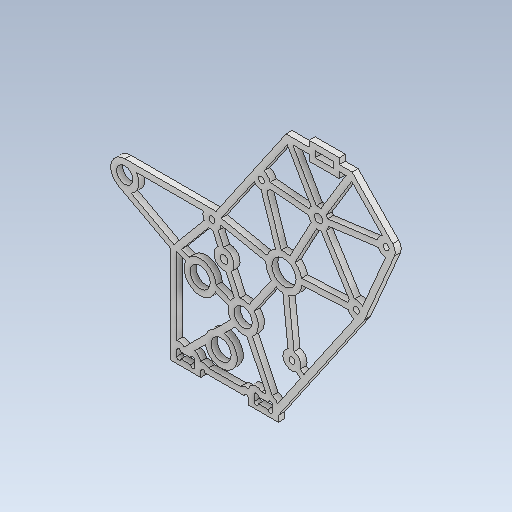
# Autodesk Inventor part: 横回転首振りフレーム２
Saved by Autodesk Inventor 2020 (Build 240168000, 168)
## iProperties
Created: 2020-02-26
Part Number: 横回転首振りフレーム２
Material: アルミニウム 2014-T4
Document SubType Name: Modeling
Designer: tanjihayato
Density: 2.8 g/cm^3
Appearance: サテン
Mass: 28.1218 g
Surface Area: 128.912 cm^2
Volume: 10.0435 cm^3
Author: tanjihayato
Autodesk Inventor part; units mm, degrees
ref_plane "YZ Plane" through (0, 0, 0) normal (1, 0, 0) x (0, 1, 0)
ref_plane "XZ Plane" through (0, 0, 0) normal (0, 1, 0) x (-1, 0, 0)
ref_plane "XY Plane" through (0, 0, 0) normal (0, 0, 1) x (1, 0, 0)
sketch "スケッチ1" plane through (0, 0, 0) normal (0, 0, 1) x (1, 0, 0)
  circle A0 centre (-11.4931, -19.1593) radius 14 construction
  circle A1 centre (16.245, -15.3385) radius 14 construction
  line L0 (-170.915, -81.4118) -> (490.0044, -81.4118)
  line L1 (-197.2268, -33.1593) -> (179.6604, -33.1593) construction
  line L2 (-178.6504, 68.5882) -> (447.0756, 68.5882) construction
  circle A2 centre (-11.4931, -19.1593) radius 14 construction
  circle A3 centre (-21.8854, 6.8407) radius 14 construction
  circle A4 centre (-0.5211, 0.3031) radius 20.05 construction
  circle A5 centre (-0.5211, 0.3031) radius 22.3421 construction
  circle A6 centre (0, 0) radius 22.3421 construction
  circle A7 centre (-0.5211, 0.3031) radius 5.05 construction
  circle A8 centre (19.689, 29.6103) radius 30.55 construction
  circle A9 centre (19.689, 29.6103) radius 10.1 construction
  circle A10 centre (39.672, 58.5882) radius 25.1 construction
  line L3 (-0.5211, 0.3031) -> (39.672, 58.5882) construction
  circle A11 centre (39.672, 58.5882) radius 27.1 construction
  circle A12 centre (19.689, 29.6103) radius 31.55 construction
  circle A13 centre (19.689, 29.6103) radius 12.1 construction
  circle A14 centre (-0.5211, 0.3031) radius 20.55 construction
  circle A15 centre (-0.5211, 0.3031) radius 6.05 construction
  circle A16 centre (36.8436, 61.4166) radius 4 construction
  circle A17 centre (36.8436, 61.4166) radius 2
  line L4 (36.8436, 61.4166) -> (39.672, 58.5882)
  line L5 (39.672, 58.5882) -> (22.909, 61.4166) construction
  circle A18 centre (22.909, 61.4166) radius 2
  circle A19 centre (22.909, 61.4166) radius 5
  line L6 (28.2635, 50.4737) -> (31.5576, 69.9968) construction
  line L7 (31.5576, 69.9968) -> (51.0806, 66.7027) construction
  line L8 (51.0806, 66.7027) -> (47.7865, 47.1796) construction
  line L9 (47.7865, 47.1796) -> (28.2635, 50.4737) construction
  circle A20 centre (39.672, 58.5882) radius 9
  circle A21 centre (28.2635, 50.4737) radius 2.5
  circle A22 centre (47.7865, 47.1796) radius 2.5
  circle A23 centre (51.0806, 66.7027) radius 2.5
  circle A24 centre (31.5576, 69.9968) radius 2.5
  circle A25 centre (28.2635, 50.4737) radius 5
  line L10 (22.909, 61.4166) -> (36.8436, 61.4166) construction
  line L11 (-26.0808, 51.4166) -> (-426.0808, 51.4166)
  line L12 (-26.0808, 24.4166) -> (23.9192, 24.4166)
  circle A26 centre (39.672, 58.5882) radius 17.5
  circle A27 centre (47.7865, 47.1796) radius 2.1
  circle A28 centre (28.2635, 50.4737) radius 2.1
  circle A29 centre (31.5576, 69.9968) radius 2.1
  circle A30 centre (51.0806, 66.7027) radius 2.1
  circle A31 centre (47.7865, 47.1796) radius 5
  circle A32 centre (31.5576, 69.9968) radius 5
  circle A33 centre (51.0806, 66.7027) radius 5
  circle A34 centre (39.672, 58.5882) radius 19.5
  circle A35 centre (39.672, 58.5882) radius 20.5
  line L13 (20.7504, 89.6882) -> (53.4998, 89.6882)
  line L14 (53.4998, 89.6882) -> (73.6516, 68.9857)
  line L15 (20.7504, 89.6882) -> (-13.977, 39.0272)
  circle A36 centre (-59.2702, 32.0272) radius 5.025 construction
  circle A37 centre (-59.2702, 32.0272) radius 4
  arc A38 (-59.2702, 39.0272) -> (-62.5897, 25.8643) centre (-59.2702, 32.0272) ccw
  line L16 (-59.2702, 39.0272) -> (-13.977, 39.0272)
  line L17 (-62.5897, 25.8643) -> (-36.5547, 11.8407)
  line L18 (-36.5547, 11.8407) -> (-36.5547, -33.1593)
  arc A39 (74.5655, 64.0796) -> (73.6516, 68.9857) centre (70.4271, 65.8469) ccw
  circle A40 centre (8.5193, 63.8863) radius 4.5 construction
  arc A41 (59.4085, 28.8085) -> (59.8353, 29.5856) centre (55.6969, 31.3528) ccw
  circle A42 centre (23.6647, -6.2198) radius 4.5
  circle A43 centre (-16.0241, 34.5272) radius 4.5 construction
  line L19 (59.8353, 29.5856) -> (74.5655, 64.0796)
  line L20 (32.172, 89.6882) -> (32.172, 92.6882)
  line L21 (32.172, 92.6882) -> (47.172, 92.6882)
  line L22 (47.172, 92.6882) -> (47.172, 89.6882)
  line L23 (35.172, 89.6882) -> (35.172, 86.6882)
  line L24 (35.172, 86.6882) -> (44.172, 86.6882)
  line L25 (44.172, 86.6882) -> (44.172, 89.6882)
  circle A44 centre (70.4271, 65.8469) radius 1.5
  circle A45 centre (55.6969, 31.3528) radius 1.5
  circle A46 centre (23.6647, -6.2198) radius 1.5
  circle A47 centre (-16.0241, 34.5272) radius 1.5
  circle A48 centre (8.5193, 63.8863) radius 1.5
  circle A49 centre (-10.0662, 20.4166) radius 4 construction
  circle A50 centre (-10.0662, 20.4166) radius 2
  line L26 (1.9305, -36.1593) -> (16.9305, -36.1593)
  line L27 (16.9305, -36.1593) -> (16.9305, -33.1593)
  line L28 (1.9305, -33.1593) -> (1.9305, -36.1593)
  arc A51 (1.9305, -33.1593) -> (-0.1695, -33.1593) centre (0.8805, -33.1593) ccw
  line L29 (13.9305, -30.1593) -> (13.9305, -33.1593)
  arc A52 (13.9305, -30.1593) -> (11.8305, -30.1593) centre (12.8805, -30.1593) ccw
  line L30 (7.0305, -30.1593) -> (11.8305, -30.1593)
  arc A53 (7.0305, -30.1593) -> (4.9305, -30.1593) centre (5.9805, -30.1593) ccw
  line L31 (4.9305, -33.1593) -> (4.9305, -30.1593)
  arc A54 (4.9305, -33.1593) -> (7.0305, -33.1593) centre (5.9805, -33.1593) ccw
  arc A55 (11.8305, -33.1593) -> (13.9305, -33.1593) centre (12.8805, -33.1593) ccw
  line L32 (-36.5547, -36.1593) -> (-21.5547, -36.1593)
  line L33 (-21.5547, -36.1593) -> (-21.5547, -33.1593)
  arc A56 (-19.4547, -33.1593) -> (-21.5547, -33.1593) centre (-20.5047, -33.1593) ccw
  line L34 (-36.5547, -33.1593) -> (-36.5547, -36.1593)
  arc A57 (-33.5547, -33.1593) -> (-31.4547, -33.1593) centre (-32.5047, -33.1593) ccw
  line L35 (-33.5547, -33.1593) -> (-33.5547, -30.1593)
  arc A58 (-31.4547, -30.1593) -> (-33.5547, -30.1593) centre (-32.5047, -30.1593) ccw
  line L36 (-31.4547, -30.1593) -> (-26.6547, -30.1593)
  arc A59 (-24.5547, -30.1593) -> (-26.6547, -30.1593) centre (-25.6047, -30.1593) ccw
  line L37 (-24.5547, -30.1593) -> (-24.5547, -33.1593)
  arc A60 (-26.6547, -33.1593) -> (-24.5547, -33.1593) centre (-25.6047, -33.1593) ccw
  line L38 (59.4085, 28.8085) -> (16.9305, -33.1593)
  circle A61 centre (-21.8854, 6.8407) radius 5
  circle A62 centre (-11.4931, -19.1593) radius 5
  line L39 (-31.4547, -33.1593) -> (-26.6547, -33.1593)
  line L40 (-19.4547, -33.1593) -> (-0.1695, -33.1593)
  line L41 (7.0305, -33.1593) -> (11.8305, -33.1593)
  line L42 (0.4485, -25.8914) -> (-27.1419, -10.3373) construction
  line L43 (-27.1419, -10.3373) -> (-17.3768, 21.5744) construction
  circle A63 centre (-21.8854, 6.8407) radius 8
  circle A64 centre (-11.4931, -19.1593) radius 8
  circle A65 centre (-19.5445, 14.4905) radius 1.3
  circle A66 centre (-24.2262, -0.8092) radius 1.3
  circle A67 centre (-18.4619, -15.2306) radius 1.3
  circle A68 centre (-4.5242, -23.088) radius 1.3
  circle A69 centre (-0.5211, 0.3031) radius 4.5
  circle A70 centre (19.689, 29.6103) radius 6
  arc A71 (87.3323, 12.0445) -> (87.1264, 18.8999) centre (85.1711, 15.4104) ccw
  line L44 (16.9305, -33.1593) -> (87.3323, 12.0445)
  line L45 (87.1264, 18.8999) -> (61.4227, 33.3027)
  circle A72 centre (85.1711, 15.4104) radius 2
  dimension "d0" = 150
  dimension "d1" = 28
  dimension "d2" = 28
  dimension "d3" = 40.1
  dimension "d4" = 10.1
  dimension "d5" = 61.1
  dimension "d6" = 20.2
  dimension "d7" = 50.2
  dimension "d8" = 10
  dimension "d9" = 2
  dimension "d10" = 1
  dimension "d11" = 2
  dimension "d12" = 0.5
  dimension "d13" = 1
  dimension "d14" = 40
  dimension "d15" = 8
  dimension "d16" = 4
  dimension "d17" = 4
  dimension "d18" = 45
  dimension "d19" = 17
  dimension "d20" = 4
  dimension "d21" = 3
  dimension "d22" = 1
  dimension "d23" = 5
  dimension "d24" = 5
  dimension "d25" = 5
  dimension "d26" = 5
  dimension "d27" = 10
  dimension "d28" = 400
  dimension "d29" = 10
  dimension "d30" = 50
  dimension "d31" = 50
  dimension "d32" = 27
  dimension "d33" = 27
  dimension "d34" = 35
  dimension "d35" = 4.2
  dimension "d36" = 4.2
  dimension "d37" = 4.2
  dimension "d38" = 4.2
  dimension "d39" = 10
  dimension "d40" = 10
  dimension "d41" = 10
  dimension "d42" = 2
  dimension "d43" = 1
  dimension "d44" = 8
  dimension "d45" = 3
  dimension "d46" = 4
  dimension "d47" = 9
  dimension "d48" = 9
  dimension "d49" = 9
  dimension "d50" = 9
  dimension "d51" = 9
  dimension "d52" = 3
  dimension "d53" = 15
  dimension "d54" = 3
  dimension "d55" = 9
  dimension "d56" = 3
  dimension "d57" = 7.5
  dimension "d58" = 3
  dimension "d59" = 3
  dimension "d60" = 3
  dimension "d61" = 3
  dimension "d62" = 3
  dimension "d63" = 8
  constraints: 90 end point, 71 centre point, 34 point on circle, 32 coincident, 23 tangent, 12 point on line, 7 perpendicular, 6 horizontal, 3 parallel, 1 collinear, 1 equal radius, 1 vertical, 22 other
  measures "d0" distance between parallel lines of L0 L2
  measures "d1" diameter of A2
  measures "d2" diameter of A3
  measures "d3" diameter of A4
  measures "d4" diameter of A7
  measures "d5" diameter of A8
  measures "d6" diameter of A9
  measures "d7" diameter of A10
  measures "d8" distance from line of L2 L3.end
  measures "d10" radial gap between concentric circles of A8 A12
  measures "d11" radial gap between concentric circles of A9 A13
  measures "d12" radial gap between concentric circles of A4 A14
  measures "d13" radial gap between concentric circles of A7 A15
  measures "d15" diameter of A16
  measures "d16" diameter of A17
  measures "d17" distance of A16.centre L3.end
  measures "d18" angle of L0 L4
  measures "d19" distance of L3.end L5.end
  measures "d20" diameter of A18
  measures "d21" radial gap between concentric circles of A18 A19
  measures "d23" diameter of A21
  measures "d24" diameter of A22
  measures "d25" diameter of A23
  measures "d26" diameter of A24
  measures "d27" diameter of A25
  measures "d28" distance of L11.start L11.end
  measures "d29" distance between parallel lines of L10 L11
  measures "d30" distance of L5.end L11.start
  measures "d31" distance of L12.start L12.end
  measures "d32" distance between parallel lines of L12 L11
  measures "d33" distance of L11.start L12.start
  measures "d34" diameter of A26
  measures "d35" diameter of A27
  measures "d36" diameter of A28
  measures "d37" diameter of A29
  measures "d38" diameter of A30
  measures "d39" diameter of A31
  measures "d40" diameter of A32
  measures "d41" diameter of A33
  measures "d42" radial gap between concentric circles of A26 A34
  measures "d43" radial gap between concentric circles of A34 A35
  measures "d44" diameter of A37
  measures "d45" radial gap between concentric circles of A37 A38
  measures "d47" diameter of A39
  measures "d48" diameter of A40
  measures "d49" diameter of A41
  measures "d50" diameter of A42
  measures "d51" diameter of A43
  measures "d52" distance of L20.start L20.end
  measures "d53" distance of L20.end L21.end
  measures "d54" distance of L23.start L23.end
  measures "d55" distance of L23.end L24.end
  measures "d56" distance between parallel lines of L22 L25
  measures "d57" distance from line of L3.end L20
  measures "d58" diameter of A44
  measures "d59" diameter of A45
  measures "d60" diameter of A46
  measures "d61" diameter of A47
  measures "d62" diameter of A48
  measures "d63" diameter of A49
extrude "押し出し1" add sketch "スケッチ1" along normal blind 3 contours A18 A26 | A18 A26 A19 | A26 A18 | A18 A26 A19 A34 | A26 A32 A20 A25 A19 | A19 A34 A26 A25 A31 A33 A32 | A34 A19 A35 | A19 A35 A34 | A32 A26 | A26 A32 | A26 A25 | A25 A26 | A35 A19 | A26 A33 A20 A32 | A20 | A20 A31 A26 A25 | A33 A26 | A26 A33 | A33 A26 A31 A20 | A31 A26 | A26 A31 | A21 | A22 | A23 | A24 | A27 | A28 | A29 | A30 | L13 L23 L24 L25 L14 A39 L19 A41 L38 L27 L26 L28 A51 L40 A56 L33 L32 L34 L18 L17 A38 L16 L15 | L20 L21 L22 L13 | A42 | A63 A66 A65 | A65 A63 | A63 A65 | A66 A63 | A63 A66 | A64 A68 A67 | A67 A64 | A64 A67 | A68 A64 | A64 A68
sketch "スケッチ2" plane through (0, 0, 3) normal (0, 0, 1) x (1, 0, 0)
  line L0 (-13.977, 39.0272) -> (-59.2702, 39.0272) projected
  arc A0 (-59.2702, 39.0272) -> (-62.5897, 25.8643) centre (-59.2702, 32.0272) ccw projected
  line L1 (-62.5897, 25.8643) -> (-36.5547, 11.8407) projected
  line L2 (-36.5547, 11.8407) -> (-36.5547, -36.1593) projected
  line L3 (-36.5547, -36.1593) -> (-21.5547, -36.1593) projected
  line L4 (-21.5547, -36.1593) -> (-21.5547, -33.1593) projected
  arc A1 (-19.4547, -33.1593) -> (-21.5547, -33.1593) centre (-20.5047, -33.1593) ccw projected
  line L5 (-19.4547, -33.1593) -> (-0.1695, -33.1593) projected
  arc A2 (1.9305, -33.1593) -> (-0.1695, -33.1593) centre (0.8805, -33.1593) ccw projected
  line L6 (1.9305, -33.1593) -> (1.9305, -36.1593) projected
  line L7 (1.9305, -36.1593) -> (16.9305, -36.1593) projected
  line L8 (16.9305, -36.1593) -> (16.9305, -33.1593) projected
  line L9 (16.9305, -33.1593) -> (59.4085, 28.8085) projected
  arc A3 (59.4085, 28.8085) -> (59.8353, 29.5856) centre (55.6969, 31.3528) ccw projected
  line L10 (59.8353, 29.5856) -> (74.5655, 64.0796) projected
  arc A4 (74.5655, 64.0796) -> (73.6516, 68.9857) centre (70.4271, 65.8469) ccw projected
  line L11 (73.6516, 68.9857) -> (53.4998, 89.6882) projected
  line L12 (53.4998, 89.6882) -> (47.172, 89.6882) projected
  line L13 (47.172, 89.6882) -> (47.172, 92.6882) projected
  line L14 (47.172, 92.6882) -> (32.172, 92.6882) projected
  line L15 (32.172, 92.6882) -> (32.172, 89.6882) projected
  line L16 (32.172, 89.6882) -> (20.7504, 89.6882) projected
  line L17 (20.7504, 89.6882) -> (-13.977, 39.0272) projected
  circle A5 centre (36.8436, 61.4166) radius 2 projected
  arc A6 (-26.6547, -33.1593) -> (-24.5547, -33.1593) centre (-25.6047, -33.1593) ccw projected
  line L18 (-26.6547, -33.1593) -> (-31.4547, -33.1593) projected
  arc A7 (-33.5547, -33.1593) -> (-31.4547, -33.1593) centre (-32.5047, -33.1593) ccw projected
  line L19 (-33.5547, -33.1593) -> (-33.5547, -30.1593) projected
  arc A8 (-31.4547, -30.1593) -> (-33.5547, -30.1593) centre (-32.5047, -30.1593) ccw projected
  line L20 (-31.4547, -30.1593) -> (-26.6547, -30.1593) projected
  arc A9 (-24.5547, -30.1593) -> (-26.6547, -30.1593) centre (-25.6047, -30.1593) ccw projected
  line L21 (-24.5547, -30.1593) -> (-24.5547, -33.1593) projected
  line L22 (13.9305, -30.1593) -> (13.9305, -33.1593) projected
  arc A10 (11.8305, -33.1593) -> (13.9305, -33.1593) centre (12.8805, -33.1593) ccw projected
  line L23 (11.8305, -33.1593) -> (7.0305, -33.1593) projected
  arc A11 (4.9305, -33.1593) -> (7.0305, -33.1593) centre (5.9805, -33.1593) ccw projected
  line L24 (4.9305, -33.1593) -> (4.9305, -30.1593) projected
  arc A12 (7.0305, -30.1593) -> (4.9305, -30.1593) centre (5.9805, -30.1593) ccw projected
  line L25 (7.0305, -30.1593) -> (11.8305, -30.1593) projected
  arc A13 (13.9305, -30.1593) -> (11.8305, -30.1593) centre (12.8805, -30.1593) ccw projected
  circle A14 centre (8.5193, 63.8863) radius 1.5 projected
  circle A15 centre (-59.2702, 32.0272) radius 4 projected
  circle A16 centre (-0.5211, 0.3031) radius 4.5 projected
  circle A17 centre (-16.0241, 34.5272) radius 1.5 projected
  circle A18 centre (70.4271, 65.8469) radius 1.5 projected
  circle A19 centre (55.6969, 31.3528) radius 1.5 projected
  circle A20 centre (-10.0662, 20.4166) radius 2 projected
  circle A21 centre (19.689, 29.6103) radius 6 projected
  line L26 (35.172, 89.6882) -> (44.172, 89.6882) projected
  line L27 (44.172, 89.6882) -> (44.172, 86.6882) projected
  line L28 (44.172, 86.6882) -> (35.172, 86.6882) projected
  line L29 (35.172, 86.6882) -> (35.172, 89.6882) projected
  circle A22 centre (-11.4931, -19.1593) radius 5 projected
  circle A23 centre (-21.8854, 6.8407) radius 5 projected
  circle A24 centre (23.6647, -6.2198) radius 1.5 projected
  line L30 (22.3311, 86.6882) -> (35.172, 86.6882)
  line L31 (35.172, 86.6882) -> (35.172, 89.6882)
  line L32 (35.172, 89.6882) -> (44.172, 89.6882)
  line L33 (44.172, 89.6882) -> (44.172, 86.6882)
  line L34 (44.172, 86.6882) -> (52.2334, 86.6882)
  line L35 (52.2334, 86.6882) -> (71.5019, 66.8931)
  arc A25 (71.8065, 65.2578) -> (71.5019, 66.8931) centre (70.4271, 65.8469) ccw
  line L36 (71.8065, 65.2578) -> (57.0763, 30.7638)
  arc A26 (56.9341, 30.5047) -> (57.0763, 30.7638) centre (55.6969, 31.3528) ccw
  line L37 (56.9341, 30.5047) -> (13.9305, -32.2298)
  line L38 (13.9305, -32.2298) -> (13.9305, -33.1593)
  line L39 (13.9305, -33.1593) -> (4.9305, -33.1593)
  arc A27 (4.9305, -33.1593) -> (-1.8402, -30.1593) centre (0.8805, -33.1593) ccw
  line L40 (-1.8402, -30.1593) -> (-17.7839, -30.1593)
  arc A28 (-17.7839, -30.1593) -> (-24.5547, -33.1593) centre (-20.5047, -33.1593) ccw
  line L41 (-24.5547, -33.1593) -> (-33.5547, -33.1593)
  line L42 (-33.5547, -33.1593) -> (-33.5547, 13.6322)
  line L43 (-33.5547, 13.6322) -> (-61.1671, 28.5055)
  arc A29 (-59.2702, 36.0272) -> (-61.1671, 28.5055) centre (-59.2702, 32.0272) ccw
  line L44 (-59.2702, 36.0272) -> (-12.3962, 36.0272)
  line L45 (-12.3962, 36.0272) -> (22.3311, 86.6882)
  line L46 (32.172, 83.6882) -> (47.172, 83.6882)
  line L47 (47.172, 83.6882) -> (47.172, 92.6882)
  line L48 (47.172, 92.6882) -> (32.172, 92.6882)
  line L49 (32.172, 92.6882) -> (32.172, 83.6882)
  circle A30 centre (8.5193, 63.8863) radius 4.5
  circle A31 centre (36.8436, 61.4166) radius 5
  circle A32 centre (70.4271, 65.8469) radius 4.5
  circle A33 centre (55.6969, 31.3528) radius 4.5
  circle A34 centre (19.689, 29.6103) radius 9
  circle A35 centre (23.6647, -6.2198) radius 4.5
  circle A36 centre (-0.5211, 0.3031) radius 7.5
  circle A37 centre (-11.4931, -19.1593) radius 8
  circle A38 centre (-21.8854, 6.8407) radius 8
  circle A39 centre (-10.0662, 20.4166) radius 5
  circle A40 centre (-16.0241, 34.5272) radius 4.5
  circle A41 centre (-59.2702, 32.0272) radius 7
  line L50 (10.1598, -27.1593) -> (8.7013, -27.1593)
  arc A42 (8.7013, -27.1593) -> (1.9305, -30.1593) centre (5.9805, -30.1593) ccw
  line L51 (1.9305, -30.1593) -> (1.9305, -33.1593)
  arc A43 (1.9305, -33.1593) -> (8.7013, -36.1593) centre (5.9805, -33.1593) ccw
  line L52 (8.7013, -36.1593) -> (10.1598, -36.1593)
  arc A44 (10.1598, -36.1593) -> (16.9305, -33.1593) centre (12.8805, -33.1593) ccw
  line L53 (16.9305, -33.1593) -> (16.9305, -30.1593)
  arc A45 (16.9305, -30.1593) -> (10.1598, -27.1593) centre (12.8805, -30.1593) ccw
  line L54 (-28.3254, -27.1593) -> (-29.7839, -27.1593)
  arc A46 (-29.7839, -27.1593) -> (-36.5547, -30.1593) centre (-32.5047, -30.1593) ccw
  line L55 (-36.5547, -30.1593) -> (-36.5547, -33.1593)
  arc A47 (-36.5547, -33.1593) -> (-29.7839, -36.1593) centre (-32.5047, -33.1593) ccw
  line L56 (-29.7839, -36.1593) -> (-28.3254, -36.1593)
  arc A48 (-28.3254, -36.1593) -> (-21.5547, -33.1593) centre (-25.6047, -33.1593) ccw
  line L57 (-21.5547, -33.1593) -> (-21.5547, -30.1593)
  arc A49 (-21.5547, -30.1593) -> (-28.3254, -27.1593) centre (-25.6047, -30.1593) ccw
  circle A50 centre (70.4271, 65.8469) radius 1.5 projected
  line L58 (36.8436, 61.4166) -> (70.4271, 65.8469) construction
  line L59 (37.0398, 59.9295) -> (70.6232, 64.3597)
  line L60 (70.2309, 67.334) -> (36.6474, 62.9037)
  arc A51 (36.6474, 62.9037) -> (37.0398, 59.9295) centre (36.8436, 61.4166) ccw
  arc A52 (70.6232, 64.3597) -> (70.2309, 67.334) centre (70.4271, 65.8469) ccw
  circle A53 centre (55.6969, 31.3528) radius 1.5 projected
  line L61 (55.6969, 31.3528) -> (36.8436, 61.4166) construction
  line L62 (56.9677, 32.1498) -> (38.1144, 62.2136)
  line L63 (35.5728, 60.6197) -> (54.4261, 30.5559)
  arc A54 (54.4261, 30.5559) -> (56.9677, 32.1498) centre (55.6969, 31.3528) ccw
  arc A55 (38.1144, 62.2136) -> (35.5728, 60.6197) centre (36.8436, 61.4166) ccw
  line L64 (8.5193, 63.8863) -> (36.8436, 61.4166) construction
  line L65 (8.389, 62.3919) -> (36.7133, 59.9223)
  line L66 (36.9739, 62.911) -> (8.6496, 65.3806)
  arc A56 (8.6496, 65.3806) -> (8.389, 62.3919) centre (8.5193, 63.8863) ccw
  arc A57 (36.7133, 59.9223) -> (36.9739, 62.911) centre (36.8436, 61.4166) ccw
  line L67 (52.2334, 86.6882) -> (36.8436, 61.4166) construction
  line L68 (50.9522, 87.4684) -> (35.5625, 62.1968)
  line L69 (38.1247, 60.6364) -> (53.5145, 85.908)
  arc A58 (53.5145, 85.908) -> (50.9522, 87.4684) centre (52.2334, 86.6882) ccw
  arc A59 (35.5625, 62.1968) -> (38.1247, 60.6364) centre (36.8436, 61.4166) ccw
  line L70 (22.3311, 86.6882) -> (36.8436, 61.4166) construction
  line L71 (21.0304, 85.9412) -> (35.5428, 60.6696)
  line L72 (38.1444, 62.1636) -> (23.6319, 87.4352)
  arc A60 (23.6319, 87.4352) -> (21.0304, 85.9412) centre (22.3311, 86.6882) ccw
  arc A61 (35.5428, 60.6696) -> (38.1444, 62.1636) centre (36.8436, 61.4166) ccw
  circle A62 centre (36.8436, 61.4166) radius 2 projected
  line L73 (36.8436, 61.4166) -> (19.689, 29.6103) construction
  line L74 (35.5234, 62.1287) -> (18.3688, 30.3224)
  line L75 (21.0092, 28.8982) -> (38.1638, 60.7046)
  arc A63 (38.1638, 60.7046) -> (35.5234, 62.1287) centre (36.8436, 61.4166) ccw
  arc A64 (18.3688, 30.3224) -> (21.0092, 28.8982) centre (19.689, 29.6103) ccw
  line L76 (8.5193, 63.8863) -> (19.689, 29.6103) construction
  line L77 (7.0931, 63.4215) -> (18.2628, 29.1455)
  line L78 (21.1152, 30.0751) -> (9.9455, 64.351)
  arc A65 (9.9455, 64.351) -> (7.0931, 63.4215) centre (8.5193, 63.8863) ccw
  arc A66 (18.2628, 29.1455) -> (21.1152, 30.0751) centre (19.689, 29.6103) ccw
  line L79 (55.6969, 31.3528) -> (19.689, 29.6103) construction
  line L80 (55.6244, 32.8511) -> (19.6165, 31.1085)
  line L81 (19.7615, 28.1121) -> (55.7694, 29.8546)
  arc A67 (55.7694, 29.8546) -> (55.6244, 32.8511) centre (55.6969, 31.3528) ccw
  arc A68 (19.6165, 31.1085) -> (19.7615, 28.1121) centre (19.689, 29.6103) ccw
  line L82 (23.6647, -6.2198) -> (19.689, 29.6103) construction
  line L83 (25.1556, -6.0544) -> (21.1799, 29.7757)
  line L84 (18.1982, 29.4449) -> (22.1739, -6.3852)
  arc A69 (22.1739, -6.3852) -> (25.1556, -6.0544) centre (23.6647, -6.2198) ccw
  arc A70 (21.1799, 29.7757) -> (18.1982, 29.4449) centre (19.689, 29.6103) ccw
  line L85 (-12.3962, 36.0272) -> (19.689, 29.6103) construction
  line L86 (-12.6904, 34.5563) -> (19.3948, 28.1394)
  line L87 (19.9832, 31.0812) -> (-12.1021, 37.498)
  arc A71 (-12.1021, 37.498) -> (-12.6904, 34.5563) centre (-12.3962, 36.0272) ccw
  arc A72 (19.3948, 28.1394) -> (19.9832, 31.0812) centre (19.689, 29.6103) ccw
  line L88 (-0.5211, 0.3031) -> (19.689, 29.6103) construction
  line L89 (0.7137, -0.5484) -> (20.9239, 28.7588)
  line L90 (18.4541, 30.4619) -> (-1.756, 1.1547)
  arc A73 (-1.756, 1.1547) -> (0.7137, -0.5484) centre (-0.5211, 0.3031) ccw
  arc A74 (20.9239, 28.7588) -> (18.4541, 30.4619) centre (19.689, 29.6103) ccw
  line L91 (-33.5547, 13.6322) -> (-0.5211, 0.3031) construction
  line L92 (-34.1159, 12.2412) -> (-1.0824, -1.0879)
  line L93 (0.0402, 1.6941) -> (-32.9934, 15.0233)
  arc A75 (-32.9934, 15.0233) -> (-34.1159, 12.2412) centre (-33.5547, 13.6322) ccw
  arc A76 (-1.0824, -1.0879) -> (0.0402, 1.6941) centre (-0.5211, 0.3031) ccw
  line L94 (-16.0241, 34.5272) -> (-33.5547, 13.6322) construction
  line L95 (-17.1733, 35.4913) -> (-34.7038, 14.5964)
  line L96 (-32.4055, 12.6681) -> (-14.875, 33.5631)
  arc A77 (-14.875, 33.5631) -> (-17.1733, 35.4913) centre (-16.0241, 34.5272) ccw
  arc A78 (-34.7038, 14.5964) -> (-32.4055, 12.6681) centre (-33.5547, 13.6322) ccw
  line L97 (-0.5211, 0.3031) -> (-16.0241, 34.5272) construction
  line L98 (0.8452, 0.922) -> (-14.6578, 35.1461)
  line L99 (-17.3905, 33.9082) -> (-1.8875, -0.3158)
  arc A79 (-1.8875, -0.3158) -> (0.8452, 0.922) centre (-0.5211, 0.3031) ccw
  arc A80 (-14.6578, 35.1461) -> (-17.3905, 33.9082) centre (-16.0241, 34.5272) ccw
  line L100 (-0.5211, 0.3031) -> (-36.5547, -36.1593) construction
  line L101 (-1.588, 1.3575) -> (-37.6216, -35.105)
  line L102 (-35.4877, -37.2137) -> (0.5458, -0.7513)
  arc A81 (0.5458, -0.7513) -> (-1.588, 1.3575) centre (-0.5211, 0.3031) ccw
  arc A82 (-37.6216, -35.105) -> (-35.4877, -37.2137) centre (-36.5547, -36.1593) ccw
  line L103 (16.9305, -36.1593) -> (-0.5211, 0.3031) construction
  line L104 (18.2835, -35.5118) -> (0.8319, 0.9507)
  line L105 (-1.8741, -0.3445) -> (15.5775, -36.8069)
  arc A83 (15.5775, -36.8069) -> (18.2835, -35.5118) centre (16.9305, -36.1593) ccw
  arc A84 (0.8319, 0.9507) -> (-1.8741, -0.3445) centre (-0.5211, 0.3031) ccw
  line L106 (23.6647, -6.2198) -> (34.3521, -15.3858) construction
  line L107 (22.6882, -7.3584) -> (33.3756, -16.5244)
  line L108 (35.3286, -14.2472) -> (24.6412, -5.0812)
  arc A85 (24.6412, -5.0812) -> (22.6882, -7.3584) centre (23.6647, -6.2198) ccw
  arc A86 (33.3756, -16.5244) -> (35.3286, -14.2472) centre (34.3521, -15.3858) ccw
  point P0 (0, 0)
  point P1 (53.6353, 63.6317)
  point P2 (46.2702, 46.3847)
  point P3 (22.6815, 62.6514)
  point P4 (44.5385, 74.0524)
  point P5 (29.5874, 74.0524)
  point P6 (28.2663, 45.5135)
  point P7 (14.1042, 46.7483)
  point P8 (37.6929, 30.4816)
  point P9 (21.6769, 11.6953)
  point P10 (3.6464, 32.8187)
  point P11 (9.5839, 14.9567)
  point P12 (-17.0379, 6.9677)
  point P13 (-24.7894, 24.0797)
  point P14 (-8.2726, 17.4151)
  point P15 (-18.5379, -17.9281)
  point P16 (8.2047, -17.9281)
  point P17 (29.0084, -10.8028)
  point P18 (53.3137, 85.5783)
  point P19 (40.6056, 64.7102)
  point P20 (41.3762, 63.5275)
  point P21 (66.0247, 66.7791)
  point P22 (68.5426, 69.9333)
  point P23 (40.6485, 58.1727)
  point P24 (54.7136, 35.7441)
  point P25 (58.7425, 34.6655)
  point P26 (70.1403, 61.356)
  point P27 (66.417, 63.8049)
  point P28 (41.7685, 60.5533)
  point P29 (28.4802, 31.5375)
  point P30 (51.3867, 32.646)
  point P31 (52.172, 34.1503)
  point P32 (38.1069, 56.5788)
  point P33 (35.8996, 56.5065)
  point P34 (25.2218, 36.7088)
  point P35 (27.8617, -7.8432)
  point P36 (29.6159, -9.3477)
  point P37 (54.5353, 27.0053)
  point P38 (51.5317, 29.6495)
  point P39 (28.6253, 28.541)
  point P40 (22.1585, 20.9557)
  point P41 (24.6877, -1.8376)
  point P42 (27.9097, -11.8366)
  point P43 (25.9086, -10.1204)
  point P44 (21.706, -2.1685)
  point P45 (19.1768, 20.6249)
  point P46 (15.886, 21.4533)
  point P47 (4.8855, 5.5011)
  point P48 (4.0044, -5.6777)
  point P49 (13.8383, -26.2242)
  point P50 (16.5397, -28.4235)
  point P51 (2.0282, -29.2754)
  point P52 (10.7479, -26.7163)
  point P53 (1.2983, -6.9728)
  point P54 (-4.6195, -5.9781)
  point P55 (-9.8985, -11.3199)
  point P56 (-19.3131, -20.8466)
  point P57 (-24.6313, -26.228)
  point P58 (-21.6523, -29.2754)
  point P59 (-29.7694, -27.1593)
  point P60 (-18.9165, -16.1772)
  point P61 (-14.5628, -11.7717)
  point P62 (-6.7533, -3.8693)
  point P63 (-7.897, 1.6618)
  point P64 (-14.3158, 4.2518)
  point P65 (-29.1318, 10.2301)
  point P66 (-33.5547, 12.0147)
  point P67 (-33.5547, -26.2478)
  point P68 (-19.9002, 32.241)
  point P69 (-20.2668, 36.0272)
  point P70 (-53.5256, 36.0272)
  point P71 (-56.1095, 25.7813)
  point P72 (-34.8753, 14.3436)
  point P73 (-4.9196, 6.3779)
  point P74 (-9.0603, 15.5188)
  point P75 (-13.0846, 24.4027)
  point P76 (-15.6399, 30.0436)
  point P77 (-17.6019, 30.3128)
  point P78 (-31.078, 14.2504)
  point P79 (-27.3029, 12.7271)
  point P80 (-13.8997, 7.3189)
  point P81 (-6.7744, 4.4439)
  point P82 (-12.9071, 31.2815)
  point P83 (-10.2489, 25.4133)
  point P84 (-6.4306, 16.984)
  point P85 (-2.1869, 7.6158)
  point P86 (2.4158, 7.2042)
  point P87 (13.4163, 23.1564)
  point P88 (10.693, 29.8797)
  point P89 (-11.5287, 34.324)
  point P90 (-11.4741, 37.3724)
  point P91 (11.2814, 32.8215)
  point P92 (15.5133, 37.583)
  point P93 (8.4077, 59.3876)
  point P94 (4.8833, 61.235)
  point P95 (11.26, 60.3172)
  point P96 (18.3656, 38.5125)
  point P97 (22.5814, 38.1329)
  point P98 (33.2592, 57.9307)
  point P99 (31.9616, 60.3366)
  point P100 (12.6156, 62.0234)
  point P101 (33.1676, 64.8058)
  point P102 (21.3899, 85.3151)
  point P103 (9.6809, 68.2338)
  point P104 (12.8762, 65.0121)
  point P105 (32.2222, 63.3253)
  point P106 (32.172, 86.6882)
  point P107 (24.0609, 86.6882)
  point P108 (35.7691, 66.2998)
  point P109 (38.0433, 66.2706)
  point P110 (50.4771, 86.6882)
  point P111 (47.172, 86.6882)
  dimension "d79" = 3
  dimension "d80" = 3
  dimension "d81" = 3
  dimension "d82" = 3
  dimension "d83" = 3
  dimension "d84" = 3
  dimension "d85" = 3
  dimension "d86" = 3
  dimension "d87" = 3
  dimension "d88" = 3
  dimension "d89" = 3
  dimension "d90" = 3
  dimension "d91" = 3
  dimension "d92" = 3
  dimension "d93" = 3
  dimension "d94" = 3
  dimension "d95" = 3
  dimension "d96" = 3
  dimension "d97" = 3
  dimension "d98" = 3
  dimension "d99" = 3
  dimension "d100" = 3
  dimension "d101" = 3
  dimension "d102" = 3
  dimension "d103" = 3
  dimension "d104" = 3
  dimension "d105" = 3
  dimension "d106" = 3
  dimension "d107" = 3
  dimension "d108" = 3
  dimension "d109" = 3
  dimension "d110" = 3
  dimension "d111" = 3
  constraints: 192 end point, 94 point on circle, 68 tangent, 59 centre point, 17 midpoint, 17 parallel, 12 concentric, 2 point on line, 37 other
  measures "d79" distance between parallel lines of L16 L30
  measures "d80" distance between parallel lines of L28 L46
  measures "d81" radial gap between concentric circles of A14 A30
  measures "d82" radial gap between concentric circles of A5 A31
  measures "d83" radial gap between concentric circles of A18 A32
  measures "d84" radial gap between concentric circles of A19 A33
  measures "d85" radial gap between concentric circles of A21 A34
  measures "d86" radial gap between concentric circles of A24 A35
  measures "d87" radial gap between concentric circles of A16 A36
  measures "d88" radial gap between concentric circles of A22 A37
  measures "d89" radial gap between concentric circles of A23 A38
  measures "d90" radial gap between concentric circles of A20 A39
  measures "d91" radial gap between concentric circles of A17 A40
  measures "d92" radial gap between concentric circles of A15 A41
  measures "d93" distance between parallel lines of L25 L50
  measures "d94" radial gap between concentric circles of A9 A49
  measures "d95" diameter of A52
  measures "d96" diameter of A55
  measures "d97" diameter of A57
  measures "d98" diameter of A59
  measures "d99" diameter of A61
  measures "d100" diameter of A64
  measures "d101" diameter of A66
  measures "d102" diameter of A68
  measures "d103" diameter of A70
  measures "d104" diameter of A72
  measures "d105" diameter of A74
  measures "d106" diameter of A76
  measures "d107" diameter of A78
  measures "d108" diameter of A80
  measures "d109" diameter of A82
  measures "d110" diameter of A84
  measures "d111" diameter of A86
extrude "押し出し2" cut sketch "スケッチ2" against normal blind 3 contours A40 L95 A75 L43 A41 L44 | L45 L71 A31 L66 A30 | A30 L77 A34 L87 L45 | A40 L99 A39 A36 L93 A38 L96 | L49 L46 L47 L34 L68 A31 L72 L30 | A30 L65 A31 L74 A34 L78 | L86 A34 L90 A36 L98 A39 A40 | L42 L92 A38 A36 L101 A37 L54 A46 | L69 L35 A32 L60 A31 | A31 L63 A33 L80 A34 L75 | A34 L84 A35 L107 L37 A45 L104 A36 L89 | A31 L59 A32 L36 A33 L62 | A34 L81 A33 L37 L108 A35 L83 | L102 A37 A36 L105 A45 L50 A42 A27 L40 A28 A49
